Autodesk Inventor part; units mm, degrees
(part 2 of 2)
  measures "d157" radius of A101
  measures "d158" radius of A107
  measures "d159" diameter of A108
  measures "d160" distance between parallel lines of L32 L68
  measures "d161" distance between parallel lines of L28 L69
  measures "d162" distance between parallel lines of L29 L70
  measures "d163" distance between parallel lines of L30 L71
  measures "d164" radius of A112
  measures "d170" distance between parallel lines of L26 L73
  measures "d171" distance between parallel lines of L29 L74
  measures "d172" radius of A117
  measures "d173" radius of A120
  measures "d174" diameter of A122
  measures "d175" distance between parallel lines of L23 L76
  measures "d176" distance between parallel lines of L27 L77
  measures "d177" distance between parallel lines of L26 L78
  measures "d178" distance between parallel lines of L25 L79
extrude "Extrusion3" cut sketch "Sketch2" against normal blind 4.7625
body "Solid1"
